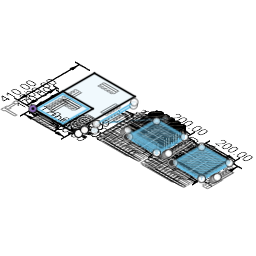
Case01 v12 (Autodesk Fusion 360 design; units mm, degrees)
Autodesk Fusion 360 part; units mm, degrees
sketch "Skizze1" plane through (0, 0, 0) normal (0, 0, 1) x (1, 0, 0)
  line L0 (0, 0) -> (200, 0)
  line L1 (200, 0) -> (200, 200)
  line L2 (200, 200) -> (0, 200)
  line L3 (0, 200) -> (0, 0)
  line L4 (15.011, 184.9717) -> (185.011, 184.9717)
  line L5 (185.011, 184.9717) -> (185.011, 14.9717)
  line L6 (185.011, 14.9717) -> (15.011, 14.9717)
  line L7 (15.011, 14.9717) -> (15.011, 184.9717)
  line L8 (0, 0) -> (270, 0)
  line L9 (270, 0) -> (270, 410)
  line L10 (270, 410) -> (0, 410)
  line L11 (0, 410) -> (0, 0)
  circle A0 centre (330, 80) radius 10
  circle A1 centre (295, 9) radius 6.5 construction
  circle A2 centre (295, 9) radius 7.5 construction
  circle A3 centre (295, 9) radius 6.5 construction
  circle A4 centre (295, 9) radius 7.5 construction
  circle A5 centre (295, 49) radius 6.5 construction
  circle A6 centre (295, 49) radius 7.5 construction
  line L12 (675, 150) -> (675, 350)
  line L13 (475, 350) -> (475, 150)
  line L14 (665, 160) -> (485, 160)
  line L15 (665, 340) -> (665, 160)
  line L16 (475, 150) -> (675, 150)
  line L17 (485, 160) -> (485, 340)
  line L18 (675, 350) -> (475, 350)
  line L19 (485, 340) -> (665, 340)
  line L20 (300, 375) -> (300, 122.1481)
  line L21 (475, 338.2551) -> (484.5108, 350)
  line L22 (475, 315.507) -> (502.9319, 350)
  line L23 (475, 292.7589) -> (521.3529, 350)
  line L24 (475, 270.0108) -> (539.774, 350)
  line L25 (475, 247.2627) -> (558.195, 350)
  line L26 (475, 224.5146) -> (576.6161, 350)
  line L27 (475, 201.7665) -> (595.0371, 350)
  line L28 (475, 179.0184) -> (613.4582, 350)
  line L29 (475, 156.2703) -> (631.8792, 350)
  line L30 (488.3435, 150) -> (650.3003, 350)
  line L31 (506.7645, 150) -> (668.7213, 350)
  line L32 (525.1856, 150) -> (675, 335.0054)
  line L33 (543.6066, 150) -> (675, 312.2573)
  line L34 (562.0277, 150) -> (675, 289.5092)
  line L35 (580.4487, 150) -> (675, 266.7611)
  line L36 (598.8698, 150) -> (675, 244.013)
  line L37 (617.2908, 150) -> (675, 221.2649)
  line L38 (635.7119, 150) -> (675, 198.5168)
  line L39 (654.1329, 150) -> (675, 175.7687)
  line L40 (672.554, 150) -> (675, 153.0206)
  line L41 (440, 170) -> (710, 170)
  line L42 (440, 175) -> (710, 175)
  line L43 (440, 180) -> (710, 180)
  line L44 (440, 185) -> (710, 185)
  line L45 (440, 190) -> (710, 190)
  line L46 (440, 195) -> (710, 195)
  line L47 (475, 210) -> (675, 210)
  line L48 (480, 155) -> (670, 155)
  line L49 (670, 155) -> (670, 345)
  line L50 (670, 345) -> (480, 345)
  line L51 (480, 345) -> (480, 155)
  line L52 (775, 224.5146) -> (876.6161, 350)
  line L53 (775, 179.0184) -> (913.4582, 350)
  line L54 (917.2908, 150) -> (975, 221.2649)
  line L55 (975, 350) -> (775, 350)
  line L56 (775, 292.7589) -> (821.3529, 350)
  line L57 (965, 160) -> (785, 160)
  line L58 (775, 247.2627) -> (858.195, 350)
  line L59 (775, 338.2551) -> (784.5108, 350)
  line L60 (785, 340) -> (965, 340)
  line L61 (775, 270.0108) -> (839.774, 350)
  line L62 (969.7566, 343.7159) -> (780.7566, 343.7159)
  line L63 (775, 315.507) -> (802.9319, 350)
  line L64 (965, 340) -> (965, 160)
  line L65 (898.8698, 150) -> (975, 244.013)
  line L66 (880.4487, 150) -> (975, 266.7611)
  line L67 (775, 156.2703) -> (931.8792, 350)
  line L68 (775, 150) -> (975, 150)
  line L69 (825.1856, 150) -> (975, 335.0054)
  line L70 (780.7566, 154.7159) -> (969.7566, 154.7159)
  line L71 (780.7566, 343.7159) -> (780.7566, 154.7159)
  line L72 (806.7645, 150) -> (968.7213, 350)
  line L73 (775, 201.7665) -> (895.0371, 350)
  line L74 (843.6066, 150) -> (975, 312.2573)
  line L75 (775, 350) -> (775, 150)
  line L76 (969.7566, 154.7159) -> (969.7566, 343.7159)
  line L77 (862.0277, 150) -> (975, 289.5092)
  line L78 (975, 150) -> (975, 350)
  line L79 (788.3435, 150) -> (950.3003, 350)
  line L80 (785, 160) -> (785, 340)
  line L81 (954.1329, 150) -> (975, 175.7687)
  line L82 (972.554, 150) -> (975, 153.0206)
  line L83 (935.7119, 150) -> (975, 198.5168)
  circle A7 centre (967.5, 157.5) radius 2
  circle A8 centre (967.5, 157.5) radius 1
  circle A9 centre (967.5, 341.5) radius 1
  circle A10 centre (967.5, 341.5) radius 2
  circle A11 centre (783, 341.5) radius 2
  circle A12 centre (783, 341.5) radius 1
  circle A13 centre (783, 157.5) radius 1
  circle A14 centre (783, 157.5) radius 2
  circle A15 centre (483, 341.5) radius 1
  circle A16 centre (483, 341.5) radius 2
  circle A17 centre (667.5, 341.5) radius 1
  circle A18 centre (667.5, 341.5) radius 2
  circle A19 centre (667.5, 157.5) radius 1
  circle A20 centre (667.5, 157.5) radius 2
  circle A21 centre (483, 157.5) radius 1
  circle A22 centre (483, 157.5) radius 2
  point P0 (475, 150)
  point P1 (775, 150)
  point P2 (1010, 190)
  point P3 (1010, 195)
  point P4 (1010, 200)
  point P5 (1010, 210)
  point P6 (1010, 205)
  point P7 (1010, 215)
  point P8 (1010, 220)
  dimension "d1" = 170
  dimension "d2" = 410
  dimension "d3" = 170
  dimension "d4" = 200
  dimension "d5" = 270
  dimension "d6" = 200
  dimension "d7" = 13
  dimension "d8" = 15
  dimension "d9" = 13
  dimension "d10" = 15
  dimension "d11" = 13
  dimension "d12" = 15
  dimension "d13" = 180
  dimension "d14" = 180
  dimension "d15" = 200
  dimension "d16" = 200
  dimension "d18" = 39
  dimension "d29" = 180
  dimension "d30" = 180
  dimension "d31" = 200
  dimension "d32" = 200
  dimension "d51" = 189
  dimension "d52" = 189
  constraint horizontal L0
  constraint vertical L1
  constraint horizontal L2
  constraint vertical L3
  constraint coincident L0.start L3.end
  constraint horizontal L4
  constraint vertical L5
  constraint horizontal L6
  constraint vertical L7
  constraint horizontal L8
  constraint vertical L9
  constraint horizontal L10
  constraint vertical L11
  constraint concentric A1 A2
  constraint concentric A3 A4
  constraint concentric A5 A6
  constraint horizontal L16
  constraint vertical L12
  constraint horizontal L18
  constraint vertical L13
  constraint coincident P0 L13.end
  constraint horizontal L19
  constraint vertical L15
  constraint horizontal L14
  constraint vertical L17
  constraint vertical L20
  constraint coincident L18 L21.end
  constraint coincident L13 L21.start
  constraint coincident L18 L22.end
  constraint coincident L18 L23.end
  constraint coincident L18 L24.end
  constraint coincident L18 L25.end
  constraint coincident L18 L26.end
  constraint coincident L18 L28.end
  constraint coincident L18 L30.end
  constraint coincident L18 L29.end
  constraint coincident L18 L27.end
  constraint coincident L18 L31.end
  constraint coincident L12 L33.end
  constraint coincident L12 L35.end
  constraint coincident L12 L37.end
  constraint coincident L12 L38.end
  constraint coincident L12 L40.end
  constraint coincident L12 L39.end
  constraint coincident L12 L36.end
  constraint coincident L12 L34.end
  constraint coincident L12 L32.end
  constraint coincident L16 L40.start
  constraint coincident L16 L39.start
  constraint coincident L16 L38.start
  constraint coincident L16 L37.start
  constraint coincident L16 L36.start
  constraint coincident L16 L35.start
  constraint coincident L16 L34.start
  constraint coincident L16 L33.start
  constraint coincident L16 L32.start
  constraint coincident L16 L31.start
  constraint coincident L16 L30.start
  constraint coincident L13 L29.start
  constraint coincident L13 L28.start
  constraint coincident L13 L27.start
  constraint coincident L13 L26.start
  constraint coincident L13 L25.start
  constraint coincident L13 L24.start
  constraint coincident L13 L23.start
  constraint coincident L13 L22.start
  constraint perpendicular L15 L41
  constraint horizontal L48
  constraint vertical L49
  constraint horizontal L50
  constraint vertical L51
  constraint horizontal L68
  constraint vertical L78
  constraint horizontal L55
  constraint vertical L75
  constraint coincident P1 L68.start
  constraint horizontal L60
  constraint vertical L64
  constraint horizontal L57
  constraint vertical L80
  constraint coincident L59.end L55
  constraint coincident L59.start L75
  constraint coincident L63.end L55
  constraint coincident L56.end L55
  constraint coincident L61.end L55
  constraint coincident L58.end L55
  constraint coincident L52.end L55
  constraint coincident L53.end L55
  constraint coincident L79.end L55
  constraint coincident L67.end L55
  constraint coincident L73.end L55
  constraint coincident L72.end L55
  constraint coincident L74.end L78
  constraint coincident L66.end L78
  constraint coincident L54.end L78
  constraint coincident L83.end L78
  constraint coincident L82.end L78
  constraint coincident L81.end L78
  constraint coincident L65.end L78
  constraint coincident L77.end L78
  constraint coincident L69.end L78
  constraint coincident L82.start L68
  constraint coincident L81.start L68
  constraint coincident L83.start L68
  constraint coincident L54.start L68
  constraint coincident L65.start L68
  constraint coincident L66.start L68
  constraint coincident L77.start L68
  constraint coincident L74.start L68
  constraint coincident L69.start L68
  constraint coincident L72.start L68
  constraint coincident L79.start L68
  constraint coincident L67.start L75
  constraint coincident L53.start L75
  constraint coincident L73.start L75
  constraint coincident L52.start L75
  constraint coincident L58.start L75
  constraint coincident L61.start L75
  constraint coincident L56.start L75
  constraint coincident L63.start L75
  constraint horizontal L70
  constraint vertical L76
  constraint horizontal L62
  constraint vertical L71
  constraint coincident L12 L47.end
  constraint coincident L13 L47.start
  measures "d1" distance of L4.start L6.end
  measures "d2" distance of L0.start L10.end
  measures "d3" distance of L5.end L6.end
  measures "d4" distance of L0.start L0.end
  measures "d5" distance of L0.start L8.end
  measures "d6" distance of L0.start L2.end
  measures "d7" diameter of A1
  measures "d8" diameter of A2
  measures "d9" diameter of A3
  measures "d10" diameter of A4
  measures "d11" diameter of A5
  measures "d12" diameter of A6
  measures "d13" distance of L14.end L17.end
  measures "d14" distance of L14.end L14.start
  measures "d15" distance of L12.start P0
  measures "d16" distance of P0 L13.start
  measures "d18" angle of L20 L21
  measures "d29" distance of L60.start L57.end
  measures "d30" distance of L57.start L57.end
  measures "d31" distance of L68.end P1
  measures "d32" distance of L55.end P1
  measures "d51" distance of L70.end L70.start
  measures "d52" distance of L70.start L62.end
extrude "Extrusion11" add sketch "Skizze1" against normal blind 49 contours L52 L58 L71 L80 | L52 L71 L73 L80 | L52 L58 L60 L80 | L52 L60 L73 L80 | L58 L61 L71 L80 | L53 L71 L73 L80 | L52 L58 L60 L62 | L52 L60 L62 L73 | L53 L60 L73 L80 | L58 L60 L61 L80 | L56 L61 L71 L80 | L53 L67 L71 L80 | L58 L60 L61 L62 | L53 L60 L62 L73 | L53 L60 L67 L80 | L56 L60 L61 L80 | L56 L63 L71 L80 | L57 L67 L70 L71 L79 L80 | L56 L60 L61 L62 | L53 L60 L62 L67 | L57 L60 L67 L79 L80 | L56 L60 L63 L80 | L60 L62 L63 L71 L80 | L56 L60 L62 L63 | L60 L62 L67 L79 | L60 L63 L80 | L57 L70 L72 L79 | L60 L62 L72 L79 | L57 L60 L72 L79 | L57 L69 L70 L72 | L60 L62 L64 L69 L72 L76 | L57 L60 L64 L69 L72 | L57 L69 L70 L74 | L57 L64 L69 L74 | L57 L70 L74 L77 | L64 L69 L74 L76 | L57 L64 L74 L77 | L57 L66 L70 L77 | L64 L74 L76 L77 | L57 L64 L66 L77 | L57 L65 L66 L70 | L64 L66 L76 L77 | L57 L64 L65 L66 | L54 L57 L65 L70 | L64 L65 L66 L76 | L54 L57 L64 L65 | L54 L57 L70 L83 | L54 L64 L65 L76 | L54 L57 L64 L83 | L57 L70 L81 L83 | L54 L64 L76 L83 | L57 L64 L81 L83 | L57 L64 L70 L76 L81 | L64 L76 L81 L83 | L57 L64 L81 | A7 | A8 | A9 | A10 | A11 | A12 | A13 | A14 makes body 1
extrude "Extrusion2" add sketch "Skizze1" along normal blind 55 separate body contours L12 L16 L40 | L12 L16 L39 L40 L41 L48 L49 | L12 L39 L41 L42 | L16 L38 L39 L48 | L12 L39 L42 | L39 L41 L42 L49 | L39 L41 L49 | L16 L37 L38 L48 | L14 L38 L39 L48 | L14 L15 L39 L48 L49 | L12 L39 L42 L43 L49 | L15 L39 L41 L49 | L15 L41 L42 L49 | L16 L36 L37 L48 | L14 L37 L38 L48 | L14 L15 L39 | L14 L15 L38 L39 L41 | L12 L43 L44 L49 | L15 L42 L43 L49 | L15 L38 L41 L42 | L16 L35 L36 L48 | L14 L36 L37 L48 | L14 L37 L38 L41 | L12 L44 L45 L49 | L15 L43 L44 L49 | L15 L38 L42 L43 | L37 L38 L41 L42 | L16 L34 L35 L48 | L14 L35 L36 L48 | L14 L36 L37 L41 | L12 L38 L45 L46 L49 | L15 L38 L44 L45 L49 | L15 L38 L43 L44 | L37 L38 L42 L43 | L36 L37 L41 L42 | L16 L33 L34 L48 | L14 L34 L35 L48 | L14 L35 L36 L41 | L12 L38 L46 | L38 L45 L49 | L15 L38 L44 | L37 L38 L43 L44 | L36 L37 L42 L43 | L35 L36 L41 L42 | L16 L32 L33 L48 | L14 L33 L34 L48 | L14 L34 L35 L41 | L12 L38 L46 L47 L49 | L38 L46 L49 | L15 L38 L45 L46 L49 | L15 L38 L45 | L15 L37 L38 L44 L45 | L36 L37 L43 L44 | L35 L36 L42 L43 | L34 L35 L41 L42 | L16 L31 L32 L48 | L14 L32 L33 L48 | L14 L33 L34 L41 | L12 L37 L47 L49 | L15 L37 L46 L47 L49 | L15 L37 L45 L46 | L36 L37 L44 L45 | L35 L36 L43 L44 | L34 L35 L42 L43 | L33 L34 L41 L42 | L16 L30 L31 L48 | L14 L31 L32 L48 | L14 L32 L33 L41 | L12 L36 L37 L49 | L37 L47 L49 | L15 L37 L46 | L36 L37 L45 L46 | L35 L36 L44 L45 | L34 L35 L43 L44 | L33 L34 L42 L43 | L32 L33 L41 L42 | L13 L16 L29 L30 L48 L51 | L14 L30 L31 L48 | L14 L31 L32 L41 | L12 L35 L36 L49 | L15 L36 L37 L47 L49 | L15 L37 L47 | L15 L36 L37 L46 L47 | L35 L36 L45 L46 | L34 L35 L44 L45 | L33 L34 L43 L44 | L32 L33 L42 L43 | L31 L32 L41 L42 | L14 L17 L29 L30 L48 L51 | L14 L30 L31 L41 | L12 L34 L35 L49 | L15 L35 L36 L49 | L15 L36 L47 | L35 L36 L46 L47 | L34 L35 L45 L46 | L33 L34 L44 L45 | L32 L33 L43 L44 | L31 L32 L42 L43 | L30 L31 L41 L42 | L13 L29 L41 L51 | L14 L17 L29 L30 L41 | L12 L33 L34 L49 | L15 L34 L35 L49 | L15 L35 L36 L47 | L34 L35 L46 L47 | L33 L34 L45 L46 | L32 L33 L44 L45 | L31 L32 L43 L44 | L30 L31 L42 L43 | L29 L30 L41 L42 | L13 L41 L42 L51 | L17 L29 L41 L51 | L12 L32 L33 L49 | L15 L33 L34 L49 | L15 L34 L35 L47 | L33 L34 L46 L47 | L32 L33 L45 L46 | L31 L32 L44 L45 | L30 L31 L43 L44 | L29 L30 L42 L43 | L17 L29 L41 L42 | L17 L29 L41 | L13 L28 L42 L43 L51 | L17 L41 L42 L51 | L12 L18 L31 L32 L49 L50 | L15 L32 L33 L49 | L15 L33 L34 L47 | L32 L33 L46 L47 | L31 L32 L45 L46 | L30 L31 L44 L45 | L29 L30 L43 L44 | L17 L29 L42 L43 | L13 L28 L43 | L17 L42 L43 L51 | L15 L19 L31 L32 L49 L50 | L15 L32 L33 L47 | L31 L32 L46 L47 | L30 L31 L45 L46 | L29 L30 L44 L45 | L17 L29 L43 L44 | L13 L28 L43 L44 | L28 L43 L44 L51 | L17 L43 L44 L51 | L18 L30 L31 L50 | L15 L19 L31 L32 L47 | L30 L31 L46 L47 | L29 L30 L45 L46 | L17 L29 L44 L45 | L13 L28 L44 L45 L51 | L28 L44 L51 | L17 L28 L44 L45 L51 | L18 L29 L30 L50 | L19 L30 L31 L50 | L19 L30 L31 L47 | L29 L30 L46 L47 | L17 L28 L29 L45 L46 | L13 L45 L46 L51 | L28 L45 L51 | L18 L28 L29 L50 | L19 L29 L30 L50 | L19 L29 L30 L47 | L28 L29 L46 L47 | L17 L28 L45 | L13 L27 L46 L51 | L17 L28 L45 L46 L51 | L18 L27 L28 L50 | L19 L28 L29 L50 | L19 L28 L29 L47 | L17 L28 L46 L47 | L17 L28 L46 | L13 L27 L47 L51 | L17 L27 L46 L47 L51 | L18 L26 L27 L50 | L19 L27 L28 L50 | L17 L19 L27 L28 L47 | L13 L26 L47 L51 | L27 L47 L51 | L18 L25 L26 L50 | L19 L26 L27 L50 | L17 L27 L47 | L13 L25 L26 L51 | L17 L26 L27 L47 L51 | L18 L24 L25 L50 | L19 L25 L26 L50 | L17 L19 L26 L27 | L13 L24 L25 L51 | L17 L25 L26 L51 | L18 L23 L24 L50 | L19 L24 L25 L50 | L17 L19 L25 L26 | L13 L23 L24 L51 | L17 L24 L25 L51 | L18 L22 L23 L50 | L19 L23 L24 L50 | L17 L19 L24 L25 | L13 L22 L23 L51 | L17 L23 L24 L51 | L18 L21 L22 L50 | L19 L22 L23 L50 | L17 L19 L23 L24 | L13 L21 L22 L51 | L17 L22 L23 L51 | L13 L18 L21 L50 L51 | L17 L19 L21 L22 L50 L51 | L17 L19 L22 L23 | L21 L50 L51 | L17 L19 L22 | A15 | A16 | A17 | A18 | A19 | A20 | A21 | A22 makes body 2
sketch "Skizze2" plane through (0, 0, 0) normal (0, 0, 1) x (1, 0, 0)
extrude "Extrusion3" add sketch "Skizze1" along normal blind 60 contours L12 L16 L40 | L12 L16 L39 L40 L41 L48 L49 | L16 L38 L39 L48 | L16 L37 L38 L48 | L14 L38 L39 L48 | L14 L15 L39 L48 L49 | L12 L39 L42 L43 L49 | L15 L39 L41 L49 | L16 L36 L37 L48 | L14 L37 L38 L48 | L14 L15 L39 | L14 L15 L38 L39 L41 | L15 L42 L43 L49 | L16 L35 L36 L48 | L14 L36 L37 L48 | L14 L37 L38 L41 | L12 L44 L45 L49 | L15 L38 L42 L43 | L16 L34 L35 L48 | L14 L35 L36 L48 | L14 L36 L37 L41 | L15 L38 L44 L45 L49 | L37 L38 L42 L43 | L16 L33 L34 L48 | L14 L34 L35 L48 | L14 L35 L36 L41 | L12 L38 L46 | L15 L38 L44 | L36 L37 L42 L43 | L16 L32 L33 L48 | L14 L33 L34 L48 | L14 L34 L35 L41 | L12 L38 L46 L47 L49 | L15 L38 L45 | L15 L37 L38 L44 L45 | L35 L36 L42 L43 | L16 L31 L32 L48 | L14 L32 L33 L48 | L14 L33 L34 L41 | L15 L37 L46 L47 L49 | L36 L37 L44 L45 | L34 L35 L42 L43 | L16 L30 L31 L48 | L14 L31 L32 L48 | L14 L32 L33 L41 | L12 L36 L37 L49 | L15 L37 L46 | L35 L36 L44 L45 | L33 L34 L42 L43 | L13 L16 L29 L30 L48 L51 | L14 L30 L31 L48 | L14 L31 L32 L41 | L15 L36 L37 L47 L49 | L15 L36 L37 L46 L47 | L34 L35 L44 L45 | L32 L33 L42 L43 | L14 L17 L29 L30 L48 L51 | L14 L30 L31 L41 | L12 L34 L35 L49 | L15 L36 L47 | L35 L36 L46 L47 | L33 L34 L44 L45 | L31 L32 L42 L43 | L13 L29 L41 L51 | L14 L17 L29 L30 L41 | L15 L34 L35 L49 | L34 L35 L46 L47 | L32 L33 L44 L45 | L30 L31 L42 L43 | L17 L29 L41 L51 | L12 L32 L33 L49 | L15 L34 L35 L47 | L33 L34 L46 L47 | L31 L32 L44 L45 | L29 L30 L42 L43 | L17 L29 L41 | L13 L28 L42 L43 L51 | L15 L32 L33 L49 | L32 L33 L46 L47 | L30 L31 L44 L45 | L17 L29 L42 L43 | L17 L42 L43 L51 | L15 L32 L33 L47 | L31 L32 L46 L47 | L29 L30 L44 L45 | L18 L30 L31 L50 | L30 L31 L46 L47 | L17 L29 L44 L45 | L13 L28 L44 L45 L51 | L17 L28 L44 L45 L51 | L19 L30 L31 L50 | L19 L30 L31 L47 | L29 L30 L46 L47 | L28 L45 L51 | L18 L28 L29 L50 | L28 L29 L46 L47 | L13 L27 L46 L51 | L19 L28 L29 L50 | L19 L28 L29 L47 | L17 L28 L46 L47 | L13 L27 L47 L51 | L17 L27 L46 L47 L51 | L18 L26 L27 L50 | L13 L26 L47 L51 | L27 L47 L51 | L19 L26 L27 L50 | L17 L26 L27 L47 L51 | L18 L24 L25 L50 | L17 L19 L26 L27 | L13 L24 L25 L51 | L19 L24 L25 L50 | L17 L24 L25 L51 | L18 L22 L23 L50 | L17 L19 L24 L25 | L13 L22 L23 L51 | L19 L22 L23 L50 | L17 L22 L23 L51 | L13 L18 L21 L50 L51 | L17 L19 L22 L23 | A19 | A20 | A21 | A22 bodies 2
extrude "Extrusion4" cut sketch "Skizze1" along normal blind 50 contours L14 L15 L39 | L14 L15 L38 L39 L41 | L15 L38 L41 L42 | L14 L37 L38 L41 | L15 L38 L42 L43 | L37 L38 L41 L42 | L14 L36 L37 L41 | L15 L38 L43 L44 | L37 L38 L42 L43 | L36 L37 L41 L42 | L14 L35 L36 L41 | L15 L38 L44 | L37 L38 L43 L44 | L36 L37 L42 L43 | L35 L36 L41 L42 | L14 L34 L35 L41 | L15 L37 L38 L44 L45 | L36 L37 L43 L44 | L35 L36 L42 L43 | L34 L35 L41 L42 | L14 L33 L34 L41 | L15 L37 L45 L46 | L36 L37 L44 L45 | L35 L36 L43 L44 | L34 L35 L42 L43 | L33 L34 L41 L42 | L14 L32 L33 L41 | L15 L37 L46 | L36 L37 L45 L46 | L35 L36 L44 L45 | L34 L35 L43 L44 | L33 L34 L42 L43 | L32 L33 L41 L42 | L14 L31 L32 L41 | L15 L36 L37 L46 L47 | L35 L36 L45 L46 | L34 L35 L44 L45 | L33 L34 L43 L44 | L32 L33 L42 L43 | L31 L32 L41 L42 | L14 L30 L31 L41 | L15 L36 L47 | L35 L36 L46 L47 | L34 L35 L45 L46 | L33 L34 L44 L45 | L32 L33 L43 L44 | L31 L32 L42 L43 | L30 L31 L41 L42 | L14 L17 L29 L30 L41 | L15 L35 L36 L47 | L34 L35 L46 L47 | L33 L34 L45 L46 | L32 L33 L44 L45 | L31 L32 L43 L44 | L30 L31 L42 L43 | L29 L30 L41 L42 | L15 L34 L35 L47 | L33 L34 L46 L47 | L32 L33 L45 L46 | L31 L32 L44 L45 | L30 L31 L43 L44 | L29 L30 L42 L43 | L17 L29 L41 L42 | L17 L29 L41 | L15 L33 L34 L47 | L32 L33 L46 L47 | L31 L32 L45 L46 | L30 L31 L44 L45 | L29 L30 L43 L44 | L17 L29 L42 L43 | L15 L32 L33 L47 | L31 L32 L46 L47 | L30 L31 L45 L46 | L29 L30 L44 L45 | L17 L29 L43 L44 | L15 L19 L31 L32 L47 | L30 L31 L46 L47 | L29 L30 L45 L46 | L17 L29 L44 L45 | L19 L30 L31 L47 | L29 L30 L46 L47 | L17 L28 L29 L45 L46 | L19 L29 L30 L47 | L28 L29 L46 L47 | L19 L28 L29 L47 | L17 L28 L46 L47 | L17 L28 L46 | L17 L19 L27 L28 L47 | L17 L19 L26 L27 | L17 L19 L25 L26 | L17 L19 L24 L25 | L17 L19 L23 L24 | L17 L19 L22 L23 | L17 L19 L22 bodies 2
extrude "Extrusion5" cut sketch "Skizze1" along normal blind 55 contours L39 L41 L42 L49 | L12 L43 L44 L49 | L12 L38 L45 L46 L49 | L12 L37 L47 L49 | L12 L35 L36 L49 | L12 L33 L34 L49 | L13 L41 L42 L51 | L12 L18 L31 L32 L49 L50 | L13 L28 L43 L44 | L28 L43 L44 L51 | L18 L29 L30 L50 | L13 L45 L46 L51 | L18 L27 L28 L50 | L18 L25 L26 L50 | L13 L25 L26 L51 | L18 L23 L24 L50 | L13 L23 L24 L51 | L18 L21 L22 L50 | L13 L21 L22 L51 bodies 2
extrude "Extrusion6" cut sketch "Skizze1" along normal blind 60 contours L13 L18 L21 L50 L51 bodies 2
extrude "Extrusion7" cut sketch "Skizze1" along normal blind 60 contours L12 L39 L41 L42 bodies 2
extrude "Extrusion8" add sketch "Skizze1" along normal blind 60 contours L12 L39 L42 bodies 2
extrude "Extrusion9" cut sketch "Skizze1" along normal blind 60 contours L38 L46 L49 bodies 2
extrude "Extrusion10" cut sketch "Skizze1" along normal blind 10 contours L14 L15 L39 L48 L49 | L14 L17 L29 L30 L48 L51 | L15 L19 L31 L32 L49 L50 | L17 L19 L21 L22 L50 L51 | A15 | A16 | A17 | A18 | A19 | A20 | A21 | A22 bodies 2
extrude "Extrusion12" cut sketch "Skizze1" 1 faces at (845.5171, 250.9344, 0) against normal blind 44 contours L52 L58 L60 L80 | L52 L60 L73 L80 | L53 L60 L73 L80 | L58 L60 L61 L80 | L53 L60 L67 L80 | L56 L60 L61 L80 | L57 L60 L67 L79 L80 | L56 L60 L63 L80 | L60 L63 L80 | L57 L60 L72 L79 | L57 L60 L64 L69 L72 | L57 L64 L69 L74 | L57 L64 L74 L77 | L57 L64 L66 L77 | L57 L64 L65 L66 | L54 L57 L64 L65 | L54 L57 L64 L83 | L57 L64 L81 L83 | L57 L64 L81 on bodies 1 bodies 1
extrude "Extrusion13" add sketch "Skizze1" against normal blind 49 contours L52 L58 L71 L80 | L52 L71 L73 L80 | L58 L61 L71 L80 | L53 L71 L73 L80 | L52 L58 L60 L62 | L52 L60 L62 L73 | L56 L61 L71 L80 | L53 L67 L71 L80 | L58 L60 L61 L62 | L53 L60 L62 L73 | L56 L63 L71 L80 | L57 L67 L70 L71 L79 L80 | L56 L60 L61 L62 | L53 L60 L62 L67 | L60 L62 L63 L71 L80 | L56 L60 L62 L63 | L60 L62 L67 L79 | L57 L70 L72 L79 | L60 L62 L72 L79 | L57 L69 L70 L72 | L60 L62 L64 L69 L72 L76 | L57 L69 L70 L74 | L57 L70 L74 L77 | L64 L69 L74 L76 | L57 L66 L70 L77 | L64 L74 L76 L77 | L57 L65 L66 L70 | L64 L66 L76 L77 | L54 L57 L65 L70 | L64 L65 L66 L76 | L54 L57 L70 L83 | L54 L64 L65 L76 | L57 L70 L81 L83 | L54 L64 L76 L83 | L57 L64 L70 L76 L81 | L64 L76 L81 L83 | A7 | A8 | A9 | A10 | A11 | A12 | A13 | A14 bodies 1
extrude "Extrusion14" cut sketch "Skizze1" along normal blind 20 contours L14 L38 L39 L48 | L15 L39 L41 L49 | L15 L41 L42 L49 | L14 L37 L38 L48 | L15 L42 L43 L49 | L14 L36 L37 L48 | L15 L43 L44 L49 | L14 L35 L36 L48 | L15 L38 L44 L45 L49 | L14 L34 L35 L48 | L38 L45 L49 | L14 L33 L34 L48 | L15 L38 L45 L46 L49 | L15 L38 L45 | L14 L32 L33 L48 | L15 L37 L46 L47 L49 | L14 L31 L32 L48 | L37 L47 L49 | L14 L30 L31 L48 | L15 L36 L37 L47 L49 | L15 L35 L36 L49 | L15 L34 L35 L49 | L17 L29 L41 L51 | L15 L33 L34 L49 | L17 L41 L42 L51 | L15 L32 L33 L49 | L17 L42 L43 L51 | L17 L43 L44 L51 | L17 L28 L44 L45 L51 | L19 L30 L31 L50 | L28 L45 L51 | L19 L29 L30 L50 | L17 L28 L45 | L17 L28 L45 L46 L51 | L19 L28 L29 L50 | L17 L27 L46 L47 L51 | L19 L27 L28 L50 | L27 L47 L51 | L19 L26 L27 L50 | L17 L27 L47 | L17 L26 L27 L47 L51 | L19 L25 L26 L50 | L17 L25 L26 L51 | L19 L24 L25 L50 | L17 L24 L25 L51 | L19 L23 L24 L50 | L17 L23 L24 L51 | L19 L22 L23 L50 | L17 L22 L23 L51 bodies 2
extrude "Extrusion15" cut sketch "Skizze1" against normal blind 39 contours L57 L67 L70 L71 L79 L80 | L60 L62 L63 L71 L80 | L60 L62 L64 L69 L72 L76 | L57 L64 L70 L76 L81 | A7 | A8 | A9 | A10 | A11 | A12 | A13 | A14 bodies 1
extrude "Extrusion16" cut sketch "Skizze1" 4 faces at (907.3664, 342.4772, 0) (968.171, 273.4934, 0) (848.8518, 156.4772, 0) (782.171, 218.2047, 0) against normal blind 29 contours L52 L58 L71 L80 | L52 L71 L73 L80 | L58 L61 L71 L80 | L53 L71 L73 L80 | L52 L58 L60 L62 | L52 L60 L62 L73 | L56 L61 L71 L80 | L53 L67 L71 L80 | L58 L60 L61 L62 | L53 L60 L62 L73 | L56 L63 L71 L80 | L56 L60 L61 L62 | L53 L60 L62 L67 | L56 L60 L62 L63 | L60 L62 L67 L79 | L57 L70 L72 L79 | L57 L69 L70 L72 | L57 L69 L70 L74 | L57 L70 L74 L77 | L64 L69 L74 L76 | L57 L66 L70 L77 | L64 L74 L76 L77 | L57 L65 L66 L70 | L64 L66 L76 L77 | L54 L57 L65 L70 | L64 L65 L66 L76 | L54 L57 L70 L83 | L54 L64 L65 L76 | L57 L70 L81 L83 | L54 L64 L76 L83 | L64 L76 L81 L83 on bodies 1 bodies 1
move_body "Verschieben1" bodies 1 to x (1, 0, 0) y (0, 1, 0) z (0, 0, 1) at (0, 0, 49)
sketch "Skizze3" plane through (0, 0, 5) normal (0, 0, 1) x (-1, 0, 0)
  line L0 (-785, -340) -> (-785, -160)
  line L1 (-785, -160) -> (-965, -160)
  line L2 (-965, -160) -> (-965, -340)
  line L3 (-965, -340) -> (-785, -340)
  line L4 (-320, -350) -> (-320, -150)
  line L5 (-320, -150) -> (-503.7876, -376.9588)
  dimension "d65" = 39
  constraint vertical L4
  measures "d65" angle of L4 L5
extrude "Extrusion17" add sketch "Skizze1" along normal blind 12 contours A7 | A10 | A11 | A14 bodies 1
extrude "Extrusion18" cut sketch "Skizze1" along normal blind 13 contours A16 | A18 | A20 | A22 bodies 2
extrude "Extrusion19" cut sketch "Skizze1" along normal blind 20 contours A8 | A9 | A12 | A13 bodies 1
extrude "Extrusion20" cut sketch "Skizze1" along normal blind 20 contours A15 | A17 | A19 | A21 bodies 2
thread "Gewinde1" "ISO Metric profile 2.0 M2x0.4 6H" major diameter 2.074 minor diameter 1.623 pitch 0.4 angle 60 resizes the face on face at (667.5249, 342.4997, 17.6667) on bodies 2
thread "Gewinde2" "ISO Metric profile 2.0 M2x0.4 6H" major diameter 2.074 minor diameter 1.623 pitch 0.4 angle 60 resizes the face on face at (483.6983, 342.2159, 15.3333) on bodies 2
thread "Gewinde3" "ISO Metric profile 2.0 M2x0.4 6H" major diameter 2.074 minor diameter 1.623 pitch 0.4 angle 60 resizes the face on face at (483.9691, 157.2532, 15.3333) on bodies 2
thread "Gewinde4" "ISO Metric profile 2.0 M2x0.4 6H" major diameter 2.074 minor diameter 1.623 pitch 0.4 angle 60 resizes the face on face at (667.5249, 158.4997, 17.6667) on bodies 2
extrude "Extrusion21" add sketch "Skizze1" along normal blind 60 contours L13 L28 L43 bodies 2
named bodies: "Deckel", "Basis"
